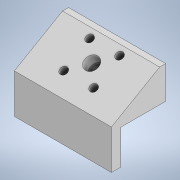
# Autodesk Inventor part: intakemount
Saved by Autodesk Inventor 2020 (Build 240168000, 168)
## iProperties
Created: 2019-12-28
Part Number: intakemount
Material: Generic
Document SubType Name: Modeling
Designer: xj82b
Density: 1 g/cm^3
Appearance: Default
Author: xj82b
Autodesk Inventor part; units mm, degrees
ref_plane "YZ Plane" through (0, 0, 0) normal (1, 0, 0) x (0, 1, 0)
ref_plane "XZ Plane" through (0, 0, 0) normal (0, 1, 0) x (-1, 0, 0)
ref_plane "XY Plane" through (0, 0, 0) normal (0, 0, 1) x (1, 0, 0)
sketch "Sketch1" plane through (0, 0, 0) normal (1, 0, 0) x (0, 1, 0)
  line L0 (0, 0) -> (0, -24)
  line L1 (0, -24) -> (20, -24)
  line L2 (20, -24) -> (20, -20.7846)
  line L3 (20, -20.7846) -> (8, 0)
  line L4 (8, 0) -> (0, 0)
  dimension "d0" = 120
  dimension "d1" = 24
  dimension "d2" = 8
  dimension "d3" = 20
  constraints: 10 end point, 2 perpendicular, 1 parallel, 1 vertical
  measures "d0" angle of L4 L3
  measures "d1" distance of L0.start L0.end
  measures "d2" distance of L3.end L0.start
  measures "d3" distance of L0.end L1.end
extrude "Extrusion1" add sketch "Sketch1" along normal blind 32
sketch "Sketch3" plane through (0, 8, 0) normal (0, 0.866, 0.5) x (1, 0, 0)
  circle A0 centre (8, 20) radius 3.6
  circle A1 centre (24, 20) radius 3.6
  circle A2 centre (24, 4) radius 3.6
  circle A3 centre (8, 4) radius 3.6
  line L0 (0, 0) -> (32, 0) projected
  line L1 (32, 24) -> (32, 0) projected
  line L2 (0, 24) -> (32, 24) projected
  circle A4 centre (16, 12) radius 3.7
  point P0 (0, -4)
  dimension "d17" = 7.2
  dimension "d18" = 7.2
  dimension "d19" = 7.2
  dimension "d20" = 7.2
  dimension "d21" = 16
  dimension "d22" = 16
  dimension "d23" = 16
  dimension "d25" = 8
  dimension "d26" = 4
  dimension "d29" = 7.4
  dimension "d30" = 8
  dimension "d31" = 8
  constraints: 5 centre point, 2 horizontal alignment, 1 vertical alignment
  measures "d17" diameter of A0
  measures "d18" diameter of A1
  measures "d19" diameter of A2
  measures "d20" diameter of A3
  measures "d21" distance of A1.centre A0.centre
  measures "d22" distance of A3.centre A2.centre
  measures "d23" distance of A2.centre A1.centre
  measures "d25" distance from line of L1 A1.centre
  measures "d26" distance from line of L2 A1.centre
  measures "d29" diameter of A4
  measures "d30" horizontal distance of A0.centre A4.centre
  measures "d31" horizontal distance of A2.centre A4.centre
extrude "Extrusion2" cut sketch "Sketch3" against normal through all contours A0 | A1 | A2 | A3
extrude "Extrusion3" cut sketch "Sketch3" against normal blind 6 contours A4
sketch "Sketch4" plane through (0, 8, 0) normal (0, 0.866, 0.5) x (1, 0, 0)
  circle A0 centre (24, 20) radius 2
  circle A1 centre (8, 20) radius 2
  circle A2 centre (24, 4) radius 2
  circle A3 centre (8, 4) radius 2
  circle A4 centre (24, 20) radius 3.6 projected
  circle A5 centre (8, 20) radius 3.6 projected
  circle A6 centre (8, 4) radius 3.6 projected
  circle A7 centre (24, 4) radius 3.6 projected
  circle A8 centre (8, 20) radius 3.6
  circle A9 centre (24, 20) radius 3.6
  circle A10 centre (24, 4) radius 3.6
  circle A11 centre (8, 4) radius 3.6
  point P0 (0, -4)
  dimension "d34" = 4
  dimension "d35" = 4
  dimension "d36" = 4
  dimension "d37" = 4
  dimension "d38" = 7.2
  dimension "d39" = 7.2
  dimension "d40" = 7.2
  dimension "d41" = 7.2
  constraints: 8 centre point, 8 concentric
  measures "d34" diameter of A0
  measures "d35" diameter of A1
  measures "d36" diameter of A2
  measures "d37" diameter of A3
  measures "d38" diameter of A8
  measures "d39" diameter of A9
  measures "d40" diameter of A10
  measures "d41" diameter of A11
extrude "Extrusion4" add sketch "Sketch4" against normal blind 6
sketch "Sketch7" plane through (0, 0, 0) normal (-1, 0, 0) x (0, 0, 1)
  line L0 (-24, 20) -> (-20.7846, 20) projected
  line L1 (-24, 20) -> (-24, 2.5)
  line L2 (-24, 0) -> (-24, 13.6308) projected
  line L3 (-24, 2.5) -> (0, 2.5)
  line L4 (-20.7846, 20) -> (0, 8) projected
  line L5 (0, 2.5) -> (0, 8)
  line L6 (0, 8) -> (-20.7846, 20)
  line L7 (-20.7846, 20) -> (-24, 20)
  point P0 (0, 0)
  dimension "d52" = 17.5
  constraints: 10 end point, 2 perpendicular, 1 collinear, 1 parallel, 1 point on line
  measures "d52" distance of L0.start L1.end
extrude "Extrusion7" add sketch "Sketch7" along normal blind 10
sketch "Sketch8" plane through (32, 0, 0) normal (1, 0, 0) x (0, 0, -1)
  line L0 (24, 20) -> (20.7846, 20) projected
  line L1 (24, 20) -> (24, 2.5)
  line L2 (24, 13.6308) -> (24, 0) projected
  line L3 (24, 2.5) -> (0, 2.5)
  line L4 (20.7846, 20) -> (0, 8) projected
  line L5 (0, 2.5) -> (0, 8)
  line L6 (0, 8) -> (20.7846, 20)
  line L7 (20.7846, 20) -> (24, 20)
  point P0 (0, 0)
  dimension "d55" = 17.5
  constraints: 10 end point, 2 perpendicular, 1 collinear, 1 parallel, 1 point on line
  measures "d55" distance of L0.start L1.end
extrude "Extrusion8" add sketch "Sketch8" along normal blind 10
sketch "Sketch9" plane through (0, 0, 0) normal (0, 0, 1) x (1, 0, 0)
  line L0 (-10, 8) -> (42, 8) projected
  line L1 (-10, 8) -> (42, 8)
  line L2 (42, 8) -> (42, -16)
  line L3 (42, -16) -> (-10, -16)
  line L4 (-10, -16) -> (-10, 8)
  point P0 (0, 0)
  dimension "d58" = 24
  dimension "d59" = 52
  constraints: 8 end point, 2 parallel, 1 horizontal, 1 perpendicular
  measures "d58" distance of L1.end L2.end
  measures "d59" distance between parallel lines of L4 L2
extrude "Extrusion9" add sketch "Sketch9" along normal blind 5
sketch "Sketch10" plane through (42, 0, 0) normal (1, 0, 0) x (0, 0, -1)
  line L0 (0, 8) -> (-8.6359, 3.0141)
  line L1 (-8.6359, 3.0141) -> (-8.6359, 11.5347)
  line L2 (-5, 8) -> (-5, -16) projected
  line L3 (-8.6359, 11.5347) -> (0, 11.5347)
  line L4 (0, 11.5347) -> (0, 8)
  line L5 (20.7846, 20) -> (0, 8) projected
  point P0 (0, 0)
  dimension "d62" = 180
  constraints: 8 end point, 2 perpendicular, 1 parallel
  measures "d62" angle of L0 L5
extrude "Extrusion10" cut sketch "Sketch10" against normal through all
body "Solid1"
